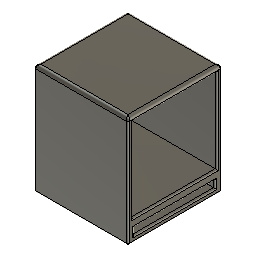
holder belt (Autodesk Fusion 360 design; units mm, degrees)
Autodesk Fusion 360 part; units mm, degrees
note: some values were not read from the file. Set by a fixed rule: which face or edge a step refers to.
sketch "Sketch3" plane through (0, 0, 0) normal (0, 0, 1) x (1, 0, 0)
  line L0 (-25, -25) -> (31, -25)
  line L1 (31, -25) -> (31, 31)
  line L2 (31, 31) -> (-25, 31)
  line L3 (-25, 31) -> (-25, -25)
  dimension "d17" = 56
  dimension "d18" = 56
  constraint perpendicular L0 L1
  constraint parallel L0 L2
  constraint parallel L1 L3
  constraint horizontal L0
  measures "d17" distance of L0.start L0.end
  measures "d18" distance of L0.start L2.end
extrude "Extrude5" add sketch "Sketch3" along normal blind 56
shell "Shell1" thickness 3 removed faces 1 at (31, -6.3333, 37.3333)
extrude "Extrude6" cut 1 faces at (-22, 11.3333, 19.6667) along direction (-1, 0, 0) blind 100
extrude "Extrude7" add 1 faces at (-6.3333, -6.3333, 0) along direction (0, 0, -1) blind 10
sketch "Sketch4" plane through (0, 0, 0) normal (1, 0, 0) x (0, 1, 0)
  line L0 (-25, -1) -> (-25, -5)
  line L1 (-25, -1) -> (-25, -5)
  line L2 (-25, -5) -> (31, -5)
  line L3 (31, -5) -> (31, -1)
  line L4 (31, -1) -> (-25, -1)
  constraint vertical L0
  constraint perpendicular L1 L2
  constraint parallel L1 L3
  constraint parallel L2 L4
extrude "Extrude8" cut sketch "Sketch4" against normal blind 37
extrude "Extrude9" cut 1 faces at (0, -6.3333, -2.3333) along direction (1, 0, 0) blind 20
extrude "Extrude10" add 1 faces at (20, -6.3333, -2.3333) along direction (-1, 0, 0) blind 5
extrude "Extrude11" add 1 faces at (15, -6.3333, -2.3333) along direction (-1, 0, 0) blind 40
sketch "Sketch5" plane through (0, 0, 0) normal (1, 0, 0) x (0, 1, 0)
  line L0 (-25, -10) -> (-25, -7)
  line L1 (-21.8343, -6.3278) -> (-21.8343, -2.3278)
  line L2 (-21.8343, -2.3278) -> (28, -2.3278)
  line L3 (28, -2.3278) -> (28, -6.3278)
  line L4 (28, -6.3278) -> (-21.8343, -6.3278)
  dimension "d34" = 3
  dimension "d35" = 4
  constraint vertical L0
  constraint perpendicular L1 L2
  constraint parallel L1 L3
  constraint parallel L2 L4
  constraint parallel L0 L1
  measures "d34" distance of L0.start L0.end
  measures "d35" distance of L1.start L1.end
extrude "Extrude12" cut sketch "Sketch5" along normal mid plane 62
sketch "Sketch6" plane through (0, 0, 0) normal (1, 0, 0) x (0, 1, 0)
extrude "Extrude13" add 1 faces at (12.3333, -21.8343, -4.5519) along direction (0, 1, 0) blind 0.528
sketch "Sketch7" plane through (0, 0, 0) normal (1, 0, 0) x (0, 1, 0)
extrude "Extrude14" add 1 faces at (12.3333, -21.3063, -4.5519) along direction (0, 1, 0) blind 0.2
extrude "Extrude15" add 1 faces at (12.3333, 28, -4.5519) along direction (0, -1, 0) blind 1
extrude "Extrude16" add 1 faces at (31, 11, 1.2241) along direction (-1, 0, 0) blind 55
fillet "Fillet4" radius 2 1 faces at (-6.3333, -6.3333, 56)
fillet "Fillet5" radius 1 1 faces at (-6.3333, -6.3333, -10)
fillet "Fillet6" radius 1 15 faces at (12.3333, -25, 14.6667) (12.3022, -24.8685, -9.4957) (-6, 12, -10) (-6, 30.1269, -9.9919) (12.3333, 31, 14.6667) (-5.6667, 29.2538, 55.9838) (-5.6667, 11.6667, 56) (11.7028, -23.2174, 55.9881) (29.2538, 11.6667, 55.9838) (31, 11, 1.2241) (30.8685, -6.3022, -9.4957) (-23.2174, 11.7028, 55.9881) (-25, 11, -8.1093) (-25, 11, 1.2241) (-24.1269, 12, -9.9919)
